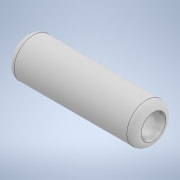
# Autodesk Inventor part: Rubber Sleeve
Saved by Autodesk Inventor 2020 (Build 240168000, 168)
## iProperties
Created: 2020-01-30
Part Number: Rubber Sleeve
Material: Generic
Document SubType Name: Modeling
Designer: cks4a449
Density: 1 g/cm^3
Appearance: Default
Author: cks4a449
Autodesk Inventor part; units mm, degrees
ref_plane "YZ Plane" through (0, 0, 0) normal (1, 0, 0) x (0, 1, 0)
ref_plane "XZ Plane" through (0, 0, 0) normal (0, 1, 0) x (-1, 0, 0)
ref_plane "XY Plane" through (0, 0, 0) normal (0, 0, 1) x (1, 0, 0)
sketch "Sketch1" plane through (0, 0, 0) normal (0, 0, 1) x (1, 0, 0)
  line L0 (0, 0) -> (113.5126, 0)
  line L1 (0, 2.3813) -> (3.9624, 2.3813)
  line L2 (3.9624, 2.3813) -> (3.9624, 0)
  line L3 (0, 0) -> (0, 2.3813)
  line L4 (0, 0) -> (0, 11.1125)
  line L5 (6.35, 17.4625) -> (107.1626, 17.4625)
  line L6 (0, 17.4625) -> (0, 11.1125)
  line L7 (3.9624, 11.1125) -> (113.5126, 11.1125)
  line L8 (0, 17.4625) -> (3.9624, 17.4625)
  line L9 (3.9624, 11.1125) -> (3.9624, 2.3813)
  arc A0 (6.35, 17.4625) -> (0, 11.1125) centre (6.35, 11.1125) ccw
  line L10 (113.5126, 11.1125) -> (113.5126, 11.1125)
  arc A1 (113.5126, 11.1125) -> (107.1626, 17.4625) centre (107.1626, 11.1125) ccw
  point P0 (113.5126, 17.4625)
  dimension "d0" = 113.5126
  dimension "d1" = 2.3813
  dimension "d2" = 3.9624
  dimension "d3" = 17.4625
  dimension "d4" = 113.5126
  dimension "d5" = 6.35
  dimension "d6" = 113.5126
  dimension "d7" = 3.9624
  dimension "d8" = 6.35
  dimension "d9" = 6.35
  constraints: 22 end point, 8 point on line, 4 perpendicular, 4 point on circle, 4 tangent, 2 centre point, 2 vertical, 1 horizontal
  measures "d0" distance of L0.start L0.end
  measures "d1" distance of L0.start L1.start
  measures "d2" distance of L1.start L1.end
  measures "d3" distance of L0.start L6.start
  measures "d4" distance of L6.start point (113.513, 17.463)
  measures "d5" distance of L6.start L6.end
  measures "d6" distance of L6.end L7.end
  measures "d7" distance of L6.start L8.end
  measures "d8" radius of A0
  measures "d9" radius of A1
revolve "Revolution1" add sketch "Sketch1" angle 360 about axis through (0, 0, 0) along (1, 0, 0) contours L4 A0 L5 A1 L7 L9 L1
body "Solid1"
